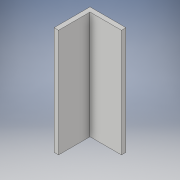
# Autodesk Inventor part: LiftAngleBracketExtension
Saved by Autodesk Inventor 2017 SP1 (Build 210196100, 196)
## iProperties
Created: 2016-08-26
Part Number: LiftAngleBracketExtension
Material: Generic
Document SubType Name: Modeling
Designer: steele
Density: 1 g/cm^3
Appearance: Default
Author: steele
Autodesk Inventor part; units mm, degrees
ref_plane "YZ Plane" through (0, 0, 0) normal (1, 0, 0) x (0, 1, 0)
ref_plane "XZ Plane" through (0, 0, 0) normal (0, 1, 0) x (-1, 0, 0)
ref_plane "XY Plane" through (0, 0, 0) normal (0, 0, 1) x (1, 0, 0)
sketch "Sketch1" plane through (0, 0, 0) normal (0, 1, 0) x (-1, 0, 0)
  line L0 (0, 0) -> (0, -50.8)
  line L1 (0, -50.8) -> (-50.8, -50.8)
  line L2 (-50.8, -50.8) -> (-50.8, -44.45)
  line L3 (-50.8, -44.45) -> (-6.35, -44.45)
  line L4 (-6.35, -44.45) -> (-6.35, 0)
  line L5 (-6.35, 0) -> (0, 0)
  dimension "d0" = 6.35
  dimension "d1" = 50.8
  constraints: 12 end point, 7 perpendicular, 1 vertical
  measures "d0" distance of L4.end L0.start
  measures "d1" distance of L0.end L1.end
extrude "Extrusion1" add sketch "Sketch1" along normal blind 152.4
body "Solid1"
